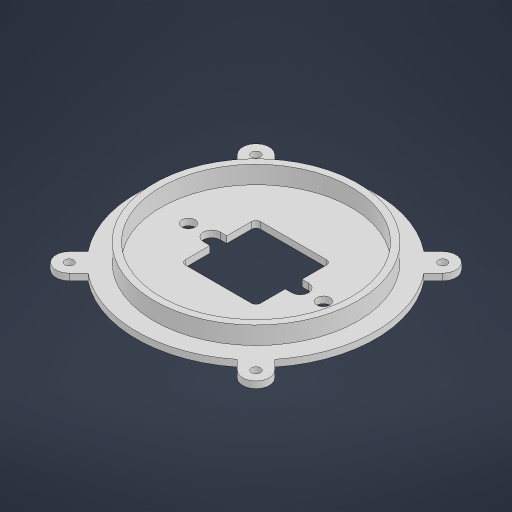
# Autodesk Inventor part: Camera_Mount
Saved by Autodesk Inventor 2024.2 (Build 282272000, 272)
## iProperties
Created: 2023-12-27
Part Number: Camera_Mount
Material: 一般
Document SubType Name: Modeling
Designer: Hanaoka
Density: 1 g/cm^3
Appearance: 既定
Author: Hanaoka
Autodesk Inventor part; units mm, degrees
ref_plane "YZ Plane" through (0, 0, 0) normal (1, 0, 0) x (0, 1, 0)
ref_plane "XZ Plane" through (0, 0, 0) normal (0, 1, 0) x (-1, 0, 0)
ref_plane "XY Plane" through (0, 0, 0) normal (0, 0, 1) x (1, 0, 0)
ref_plane "作業平面1" through (68.5489, -4.2228, -98.0091) normal (0, 1, 0) x (1, 0, 0)
sketch "スケッチ1" plane through (68.5489, -4.2228, -98.0091) normal (0, 1, 0) x (1, 0, 0)
  line L0 (9.655, 16.755) -> (9.655, 15.8775) projected
  arc A0 (6.855, 15.8775) -> (9.655, 15.8775) centre (8.255, 8.255) ccw projected
  line L1 (6.855, 15.8775) -> (6.855, 16.755) projected
  line L2 (6.855, 16.755) -> (0.755, 16.755) projected
  arc A1 (0.755, 16.755) -> (-0.245, 15.755) centre (0.755, 15.755) ccw projected
  line L3 (-0.245, 15.755) -> (-0.245, 10.155) projected
  line L4 (-0.245, 10.155) -> (-1.745, 10.155) projected
  arc A2 (-1.745, 10.155) -> (-1.745, 6.355) centre (-1.745, 8.255) ccw projected
  line L5 (-1.745, 6.355) -> (-0.245, 6.355) projected
  line L6 (-0.245, 6.355) -> (-0.245, 0.755) projected
  arc A3 (-0.245, 0.755) -> (0.755, -0.245) centre (0.755, 0.755) ccw projected
  line L7 (0.755, -0.245) -> (15.755, -0.245) projected
  arc A4 (15.755, -0.245) -> (16.755, 0.755) centre (15.755, 0.755) ccw projected
  line L8 (16.755, 0.755) -> (16.755, 6.355) projected
  line L9 (16.755, 6.355) -> (18.255, 6.355) projected
  arc A5 (18.255, 6.355) -> (18.255, 10.155) centre (18.255, 8.255) ccw projected
  line L10 (18.255, 10.155) -> (16.755, 10.155) projected
  line L11 (16.755, 10.155) -> (16.755, 15.755) projected
  arc A6 (16.755, 15.755) -> (15.755, 16.755) centre (15.755, 15.755) ccw projected
  line L12 (15.755, 16.755) -> (9.655, 16.755) projected
  circle A7 centre (-1.745, 8.255) radius 0.9 projected
  circle A8 centre (18.255, 8.255) radius 0.9 projected
  circle A9 centre (23.495, 8.255) radius 1.5 projected
  circle A10 centre (-6.985, 8.255) radius 1.5 projected
  circle A11 centre (8.255, 8.255) radius 27
  line L13 (6.855, 16.755) -> (9.655, 16.755)
  circle A12 centre (29.35, 29.35) radius 2 construction
  circle A13 centre (29.35, 29.35) radius 1
  arc A14 (31.4713, 27.2287) -> (27.2287, 31.4713) centre (29.35, 29.35) ccw
  line L14 (27.2287, 31.4713) -> (25.1073, 29.35)
  line L15 (31.4713, 27.2287) -> (29.35, 25.1073)
  line L16 (-12.84, -12.84) -> (29.35, -12.84) construction
  line L17 (29.35, -12.84) -> (29.35, 29.35) construction
  line L18 (29.35, 29.35) -> (-12.84, 29.35) construction
  line L19 (-12.84, 29.35) -> (-12.84, -12.84) construction
  line L20 (-12.84, -12.84) -> (29.35, 29.35) construction
  line L21 (29.35, -12.84) -> (-12.84, 29.35) construction
  line L22 (-14.9613, 27.2287) -> (-12.84, 25.1073)
  arc A15 (-10.7187, 31.4713) -> (-14.9613, 27.2287) centre (-12.84, 29.35) ccw
  line L23 (-10.7187, 31.4713) -> (-8.5973, 29.35)
  circle A16 centre (-12.84, 29.35) radius 2 construction
  circle A17 centre (-12.84, 29.35) radius 1
  line L24 (-10.7187, -14.9613) -> (-8.5973, -12.84)
  arc A18 (-14.9613, -10.7187) -> (-10.7187, -14.9613) centre (-12.84, -12.84) ccw
  line L25 (-14.9613, -10.7187) -> (-12.84, -8.5973)
  circle A19 centre (-12.84, -12.84) radius 2 construction
  circle A20 centre (-12.84, -12.84) radius 1
  line L26 (31.4713, -10.7187) -> (29.35, -8.5973)
  arc A21 (27.2287, -14.9613) -> (31.4713, -10.7187) centre (29.35, -12.84) ccw
  line L27 (27.2287, -14.9613) -> (25.1073, -12.84)
  circle A22 centre (29.35, -12.84) radius 2 construction
  circle A23 centre (29.35, -12.84) radius 1
  point P0 (-68.5489, -98.0091)
  point P1 (-8.5973, -12.84)
  point P2 (-12.84, -8.5973)
  point P3 (29.35, -8.5973)
  point P4 (25.1073, -12.84)
  point P5 (-12.84, 25.1073)
  point P6 (-8.5973, 29.35)
  dimension "d0" = 54
  dimension "d7" = 2
  dimension "d8" = 4
  dimension "d9" = 3
  dimension "d10" = 3
  dimension "d13" = 360
  constraints: 30 end point, 13 centre point, 11 coincident, 10 point on circle, 4 parallel, 2 midpoint, 2 tangent, 1 collinear, 1 horizontal, 1 perpendicular, 49 other
  measures "d0" diameter of A11
  measures "d7" diameter of A13
  measures "d8" diameter of A12
  measures "d9" radius of A14
  measures "d10" distance of L15.start L15.end
extrude "押し出し1" add sketch "スケッチ1" along normal blind 1.5 contours A11 | A11 L14 A14 L15 | L26 A21 L27 A11 | A11 L22 A15 L23 | L24 A18 L25 A11
sketch "スケッチ2" plane through (76.8039, -2.7228, -106.2641) normal (0, 1, 0) x (1, 0, 0)
  circle A0 centre (0, 0) radius 23
  circle A1 centre (0, 0) radius 21.5
  arc A2 (-16.8523, -21.095) -> (-21.095, -16.8523) centre (0, 0) ccw projected
  point P0 (-76.8039, -106.2641)
  dimension "d3" = 46
  dimension "d4" = 1.5
  constraints: 2 centre point, 2 coincident
  measures "d3" diameter of A0
  measures "d4" radial gap between concentric circles of A0 A1
extrude "押し出し2" add sketch "スケッチ2" along normal blind 4
